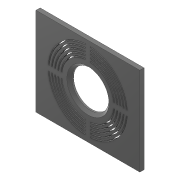
# Autodesk Inventor part: Eihalter
Saved by Autodesk Inventor 2020 (Build 240168000, 168)
## iProperties
Created: 2021-09-17
Part Number: Eihalter
Material: Acetalharz, Schwarz
Document SubType Name: Modeling
Designer: Julian Uhl
Density: 1.425 g/cm^3
Appearance: Glatt - Schwarz
Author: Julian Uhl
Autodesk Inventor part; units mm, degrees
ref_plane "YZ Plane" through (0, 0, 0) normal (1, 0, 0) x (0, 1, 0)
ref_plane "XZ Plane" through (0, 0, 0) normal (0, 1, 0) x (-1, 0, 0)
ref_plane "XY Plane" through (0, 0, 0) normal (0, 0, 1) x (1, 0, 0)
sketch "Skizze1" plane through (0, 0, 0) normal (0, 0, 1) x (1, 0, 0)
  line L0 (-72.2968, 0) -> (67.7032, 0) projected
  line L1 (0, -68.1366) -> (0, 50.8634) projected
  line L2 (-52.2968, 33.8634) -> (47.7032, 33.8634)
  line L3 (47.7032, 33.8634) -> (47.7032, -51.1366)
  line L4 (47.7032, -51.1366) -> (-52.2968, -51.1366)
  line L5 (-52.2968, -51.1366) -> (-52.2968, 33.8634)
  point P0 (0, 0)
  dimension "d0" = 100
  dimension "d1" = 85
  constraints: 8 end point, 2 parallel, 1 horizontal, 1 perpendicular
  measures "d0" distance of L2.start L2.end
  measures "d1" distance of L2.end L3.end
extrude "Extrusion1" add sketch "Skizze1" along normal blind 4
sketch "Skizze2" plane through (0, 0, 4) normal (0, 0, 1) x (1, 0, 0)
  line L0 (-52.2968, 33.8634) -> (-52.2968, -51.1366) projected
  line L1 (-52.2968, -51.1366) -> (47.7032, -51.1366) projected
  circle A0 centre (-2.2968, -8.1366) radius 17.7444
  point P0 (0, 0)
  dimension "d4" = 50
  dimension "d5" = 43
  constraints: 1 centre point, 1 coincident
  measures "d4" distance from line of L0 point (-2.297, -8.137)
  measures "d5" distance from line of L1 point (-2.297, -8.137)
extrude "Extrusion2" cut sketch "Skizze2" against normal blind 1000
chamfer "Fase1" distance 2.5 angle 45 1 edges at (-20.0412, -8.1366, 4)
sketch "Skizze3" plane through (0, 0, 4) normal (0, 0, 1) x (1, 0, 0)
  circle A0 centre (-2.2968, -8.1366) radius 17.7444 projected
  circle A1 centre (-2.2968, -8.1366) radius 25
  circle A2 centre (-2.2968, -8.1366) radius 26
  circle A3 centre (-2.2968, -8.1366) radius 28
  circle A4 centre (-2.2968, -8.1366) radius 29
  circle A5 centre (-2.2968, -8.1366) radius 31
  circle A6 centre (-2.2968, -8.1366) radius 32
  circle A7 centre (-2.2968, -8.1366) radius 34
  circle A8 centre (-2.2968, -8.1366) radius 35
  circle A9 centre (-2.2968, -8.1366) radius 37
  circle A10 centre (-2.2968, -8.1366) radius 38
  point P0 (0, 0)
  dimension "d11" = 50
  dimension "d12" = 52
  dimension "d13" = 56
  dimension "d14" = 58
  dimension "d15" = 62
  dimension "d16" = 64
  dimension "d17" = 68
  dimension "d18" = 70
  dimension "d21" = 74
  dimension "d22" = 76
  constraints: 10 centre point, 10 coincident
  measures "d11" diameter of A1
  measures "d12" diameter of A2
  measures "d13" diameter of A3
  measures "d14" diameter of A4
  measures "d15" diameter of A5
  measures "d16" diameter of A6
  measures "d17" diameter of A7
  measures "d18" diameter of A8
  measures "d21" diameter of A9
  measures "d22" diameter of A10
extrude "Extrusion3" cut sketch "Skizze3" against normal blind 1000 contours A2 | A4 | A6 | A8 | A10
sketch "Skizze4" plane through (0, 0, 4) normal (0, 0, 1) x (1, 0, 0)
  circle A0 centre (-2.2968, -8.1366) radius 17.7444 projected
  line L0 (0.2032, -8.1366) -> (-4.7968, -8.1366)
  line L1 (-4.7968, -8.1366) -> (-4.7968, -48.1366)
  line L2 (-4.7968, -48.1366) -> (0.2032, -48.1366)
  line L3 (0.2032, -48.1366) -> (0.2032, -8.1366)
  line L4 (-4.7968, -8.1366) -> (0.2032, -8.1366)
  line L5 (0.2032, -8.1366) -> (0.2032, 31.8634)
  line L6 (0.2032, 31.8634) -> (-4.7968, 31.8634)
  line L7 (-4.7968, 31.8634) -> (-4.7968, -8.1366)
  line L8 (-4.7968, -10.6366) -> (-43.2968, -10.6366)
  line L9 (-43.2968, -10.6366) -> (-43.2968, -5.6366)
  line L10 (-43.2968, -5.6366) -> (-4.7968, -5.6366)
  line L11 (-4.7968, -5.6366) -> (-4.7968, -10.6366)
  line L12 (0.2032, -10.6366) -> (40.2032, -10.6366)
  line L13 (40.2032, -10.6366) -> (40.2032, -5.6366)
  line L14 (40.2032, -5.6366) -> (0.2032, -5.6366)
  line L15 (0.2032, -5.6366) -> (0.2032, -10.6366)
  circle A1 centre (-2.2968, -8.1366) radius 17.7444
  point P0 (0, 0)
  point P1 (0.2032, -25.704)
  point P2 (-4.7968, -25.704)
  point P3 (15.2706, -5.6366)
  point P4 (15.2706, -10.6366)
  point P5 (-4.7968, 9.4307)
  point P6 (0.2032, 9.4307)
  point P7 (-19.8642, -10.6366)
  point P8 (-19.8642, -5.6366)
  dimension "d23" = 40
  dimension "d24" = 5
  dimension "d25" = 2.5
  dimension "d26" = 0
  dimension "d27" = 40
  dimension "d28" = 38.5
  dimension "d29" = 5
  dimension "d30" = 2.5
  dimension "d31" = 40
  dimension "d32" = 5
  constraints: 32 end point, 8 parallel, 4 horizontal, 4 perpendicular, 2 coincident, 2 point on line, 1 centre point, 1 concentric
  measures "d23" distance between parallel lines of L2 L0
  measures "d24" distance between parallel lines of L3 L1
  measures "d25" distance from line of L1 A0.centre
  measures "d26" distance from line of A0.centre L0
  measures "d27" distance of L5.end L4.end
  measures "d28" distance of L9.end L10.end
  measures "d29" distance between parallel lines of L10 L8
  measures "d30" distance from line of L10 A0.centre
  measures "d31" distance of L14.end L13.end
  measures "d32" distance of L13.end L12.end
extrude "Extrusion4" add sketch "Skizze4" against normal blind 4 contours A0 L14 L13 L12 | A0 L7 L6 L5 | L3 L2 L1 A0 | A0 L8 L9 L10
chamfer "Fase2" distance 2.5 angle 45 4 edges at (-2.2968, -25.881, 4) (-20.0412, -8.1366, 4) (-2.2968, 9.6077, 4) (15.4476, -8.1366, 4)
sketch "Skizze5" plane through (0, 0, 4) normal (0, 0, 1) x (1, 0, 0)
  line L0 (-52.1968, 33.7634) -> (47.6032, 33.7634)
  line L1 (47.6032, 33.7634) -> (47.6032, -51.0366)
  line L2 (47.6032, -51.0366) -> (-52.1968, -51.0366)
  line L3 (-52.1968, -51.0366) -> (-52.1968, 33.7634)
  line L4 (47.7032, 33.8634) -> (-52.2968, 33.8634) projected
  line L5 (47.7032, -51.1366) -> (47.7032, 33.8634) projected
  line L6 (-52.2968, -51.1366) -> (47.7032, -51.1366) projected
  line L7 (-52.2968, 33.8634) -> (-52.2968, -51.1366) projected
  point P0 (0, 0)
  dimension "d38" = 0.1
  dimension "d39" = 0.1
  dimension "d40" = 0.1
  dimension "d41" = 0.1
  constraints: 8 end point, 2 parallel, 1 horizontal, 1 perpendicular
  measures "d38" distance between parallel lines of L4 L0
  measures "d39" distance between parallel lines of L5 L1
  measures "d40" distance between parallel lines of L6 L2
  measures "d41" distance between parallel lines of L7 L3
extrude "Extrusion5" cut sketch "Skizze5" against normal blind 10
